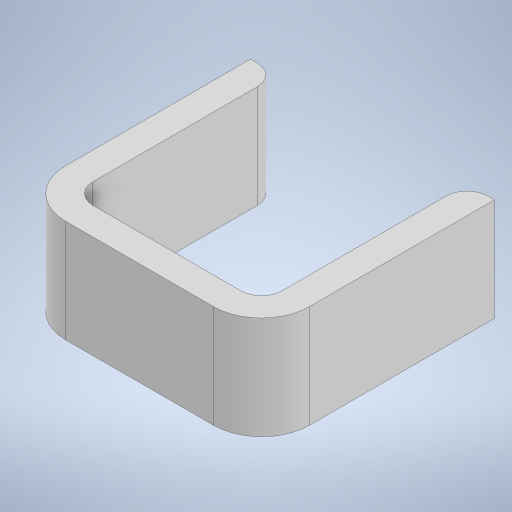
# Autodesk Inventor part: PinzaEscritorio
Saved by Autodesk Inventor 2024 (Build 280153000, 153)
## iProperties
Created: 2025-02-01
Part Number: PinzaEscritorio
Material: Genérico
Document SubType Name: Modeling
Designer: sergi
Density: 1 g/cm^3
Appearance: Valor por defecto
Author: sergi
Autodesk Inventor part; units mm, degrees
ref_plane "YZ Plane" through (0, 0, 0) normal (1, 0, 0) x (0, 1, 0)
ref_plane "XZ Plane" through (0, 0, 0) normal (0, 1, 0) x (-1, 0, 0)
ref_plane "XY Plane" through (0, 0, 0) normal (0, 0, 1) x (1, 0, 0)
sketch "Boceto1" plane through (0, 0, 0) normal (0, 1, 0) x (-1, 0, 0)
  line L0 (-3, 0) -> (-24.6, 0)
  line L1 (-27.6, -3) -> (-27.6, -27)
  line L2 (-30.6, -30) -> (-31.6, -30)
  line L3 (-31.6, -30) -> (-31.6, -3)
  line L4 (-24.6, 4) -> (-3, 4)
  line L5 (4, -3) -> (4, -30)
  line L6 (4, -30) -> (3, -30)
  line L7 (0, -27) -> (0, -3)
  arc A0 (0, -3) -> (-3, 0) centre (-3, -3) ccw
  arc A1 (-24.6, 0) -> (-27.6, -3) centre (-24.6, -3) ccw
  arc A2 (-30.6, -30) -> (-27.6, -27) centre (-30.6, -27) ccw
  arc A3 (0, -27) -> (3, -30) centre (3, -27) ccw
  arc A4 (4, -3) -> (-3, 4) centre (-3, -3) ccw
  arc A5 (-24.6, 4) -> (-31.6, -3) centre (-24.6, -3) ccw
  point P0 (0, 0)
  point P1 (-27.6, 0)
  point P2 (-27.6, -30)
  point P3 (-31.6, 4)
  point P4 (4, 4)
  point P5 (0, -30)
  dimension "d0" = 27.6
  dimension "d1" = 30
  dimension "d2" = 4
  dimension "d3" = 34
  dimension "d4" = 35.6
  dimension "d5" = 3
  dimension "d6" = 3
  dimension "d7" = 7
  constraints: 16 end point, 14 point on line, 12 point on circle, 12 tangent, 6 centre point, 6 perpendicular, 3 equal radius, 1 horizontal
  measures "d0" distance of point (0, 0) point (-27.6, 0)
  measures "d1" distance of point (-27.6, 0) point (-27.6, -30)
  measures "d2" distance of point (-27.6, -30) L2.end
  measures "d3" distance of L2.end point (-31.6, 4)
  measures "d4" distance of point (-31.6, 4) point (4, 4)
  measures "d5" radius of A0
  measures "d6" radius of A3
  measures "d7" radius of A4
extrude "Extrusión1" add sketch "Boceto1" along normal blind 15
